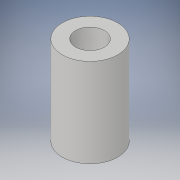
# Autodesk Inventor part: axis_left
Saved by Autodesk Inventor 2019 (Build 230136000, 136)
## iProperties
Created: 2020-10-26
Part Number: axis_left
Material: Genérico
Document SubType Name: Modeling
Designer: Juan M. Casillas
Density: 1 g/cm^3
Appearance: Valor por defecto
Author: Juan M. Casillas
## iProperties of the stored document axis_left_3DPrint.ipt
Created: 2020-10-26
Part Number: axis_left_3DPrint
Material: Genérico
Document SubType Name: Modeling
Designer: Juan M. Casillas
Density: 1 g/cm^3
Appearance: Valor por defecto
Author: Juan M. Casillas
Autodesk Inventor part; units mm, degrees
ref_plane "YZ Plane" through (0, 0, 0) normal (1, 0, 0) x (0, 1, 0)
ref_plane "XZ Plane" through (0, 0, 0) normal (0, 1, 0) x (-1, 0, 0)
ref_plane "XY Plane" through (0, 0, 0) normal (0, 0, 1) x (1, 0, 0)
sketch "Sketch1" plane through (0, 0, 0) normal (0, 1, 0) x (-1, 0, 0)
  circle A0 centre (0, 0) radius 2.6
  circle A1 centre (0, 0) radius 5
  dimension "d0" = 5.2
  dimension "d1" = 10
  constraints: 2 centre point, 2 coincident
  measures "d0" diameter of A0
  measures "d1" diameter of A1
extrude "Extrusion1" add sketch "Sketch1" along normal blind 16
body "Solid1"
